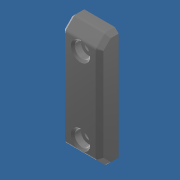
# Autodesk Inventor part: Flame_Cover_A
Saved by Autodesk Inventor 2020 (Build 240168000, 168)
## iProperties
Created: 2021-05-20
Part Number: Flame_Cover_A
Material: 一般
Document SubType Name: Modeling
Designer: ken113
Density: 1 g/cm^3
Appearance: 滑らか - 黒
Author: ken113
Autodesk Inventor part; units mm, degrees
ref_plane "YZ Plane" through (0, 0, 0) normal (1, 0, 0) x (0, 1, 0)
ref_plane "XZ Plane" through (0, 0, 0) normal (0, 1, 0) x (-1, 0, 0)
ref_plane "XY Plane" through (0, 0, 0) normal (0, 0, 1) x (1, 0, 0)
sketch "スケッチ1" plane through (0, 0, 0) normal (0, 0, 1) x (1, 0, 0)
  line L0 (-10, -30) -> (10, -30)
  line L1 (10, -30) -> (10, 30)
  line L2 (10, 30) -> (-10, 30)
  line L3 (-10, 30) -> (-10, -30)
  line L4 (-10, -30) -> (10, 30) construction
  line L5 (10, -30) -> (-10, 30) construction
  point P0 (0, 0)
  dimension "d0" = 20
  dimension "d1" = 60
  constraints: 12 end point, 2 midpoint, 2 parallel, 1 horizontal, 1 perpendicular
  measures "d0" distance of L1.end L2.end
  measures "d1" distance of L2.end L0.start
extrude "押し出し1" add sketch "スケッチ1" along normal blind 10
chamfer "面取り1" distance 5 angle 45 2 edges at (0, 30, 10) (0, -30, 10)
fillet "フィレット1" radius 2 4 edges at (0, 30, 5) (0, 25, 10) (0, -25, 10) (0, -30, 5)
chamfer "面取り2" distance 2 angle 45 18 edges at (10, 0, 10) (10, 24.9369, 9.8478) (10, 27.5, 7.5) (10, 29.8478, 4.9369) (10, 30, 2.0858) (10, -24.9369, 9.8478) (10, -27.5, 7.5) (10, -29.8478, 4.9369) (10, -30, 2.0858) (-10, 0, 10) (-10, -24.9369, 9.8478) (-10, -27.5, 7.5) (-10, -29.8478, 4.9369) (-10, -30, 2.0858) (-10, 24.9369, 9.8478) (-10, 27.5, 7.5) (-10, 29.8478, 4.9369) (-10, 30, 2.0858)
sketch "スケッチ2" plane through (0, 0, 10) normal (0, 0, 1) x (1, 0, 0)
  line L0 (-8, -24.1716) -> (-8, 24.1716) projected
  line L1 (8, -24.1716) -> (-8, -24.1716) projected
  line L2 (8, 24.1716) -> (8, -24.1716) projected
  line L3 (-8, 24.1716) -> (8, 24.1716) projected
  point P0 (0, 0)
  point P1 (0, 20)
  point P2 (0, -20)
  dimension "d11" = 40
  dimension "d12" = 20
  measures "d11" distance of point (0, -20) point (0, 20)
  measures "d12" distance of point (0, 20) point (0, 0)
hole "穴1" at (0, 20, 10) at (0, -20, 10) direction (0, 0, -1) diameter 4.2 depth 21.5 counterbore diameter 8 counterbore depth 4.2
chamfer "面取り3" distance 1 angle 45 2 edges at (0, 24, 10) (0, -16, 10)
equation "\"d12\" = 0.5 * d11"
